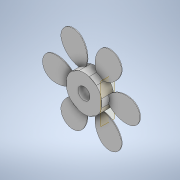
# Autodesk Inventor part: Fan
Saved by Autodesk Inventor 2022 (Build 260153000, 153)
## iProperties
Created: 2021-07-12
Part Number: Fan
Material: Generic
Document SubType Name: Modeling
Designer: Mike
Density: 1 g/cm^3
Appearance: Default
Author: Mike
Autodesk Inventor part; units mm, degrees
ref_plane "XZ Plane" through (0, 0, 0) normal (0, 1, 0) x (-1, 0, 0)
ref_plane "XY Plane" through (0, 0, 0) normal (0, 0, 1) x (1, 0, 0)
sketch "Sketch1" plane through (0, 0, 0) normal (0, 0, 1) x (1, 0, 0)
  circle A0 centre (0, 0) radius 7.5
  circle A1 centre (0, 0) radius 2.5
  dimension "d0" = 15
  dimension "d1" = 5
  constraints: 2 centre point, 2 coincident
  measures "d0" diameter of A0
  measures "d1" diameter of A1
extrude "Extrusion1" add sketch "Sketch1" against normal blind 5
ref_plane "Work Plane1" through (7.3, 0, 0) normal (1, 0, 0) x (0, 1, 0)
sketch "Sketch2" plane through (7.3, 0, 0) normal (1, 0, 0) x (0, 1, 0)
  line L0 (1.7003, -3.2966) -> (-1.6964, -3.2966)
  line L1 (-1.6964, -3.2966) -> (-1.6964, -3.0015)
  line L2 (-1.6964, -3.0015) -> (1.7003, -3.0015)
  line L3 (1.7003, -3.0015) -> (1.7003, -3.2966)
  point P0 (0, 0)
  dimension "d5" = 3.3967
  dimension "d6" = 0.2951
  dimension "d7" = 1.7003
  dimension "d8" = 3.0015
  constraints: 8 end point, 2 parallel, 1 horizontal, 1 perpendicular
  measures "d5" distance between parallel lines of L3 L1
  measures "d6" distance between parallel lines of L0 L2
  measures "d7" distance from line of point (0, 0) L3
  measures "d8" distance from line of point (0, 0) L2
extrude "Extrusion2" add sketch "Sketch2" along normal blind 20
sketch "Sketch3" plane through (7.3047, 1.7003, -3.0015) normal (0, 1, 0) x (1, 0, 0)
  line L0 (19.9953, 0) -> (19.9953, 0.2951) projected
  line L1 (-0.0143, 0) -> (19.9953, 0)
  line L2 (19.9953, 0) -> (19.9953, 0.2951)
  line L3 (19.9953, 0.2951) -> (-0.0143, 0.2951)
  line L4 (-0.0143, 0.2951) -> (-0.0143, 0)
  point P0 (-7.3047, -3.0015)
  constraints: 8 end point, 2 parallel, 1 horizontal, 1 perpendicular
extrude "Extrusion3" add sketch "Sketch3" along normal blind 10 and the other way blind 20
sketch "Sketch4" plane through (27.3, 11.7003, -3.2966) normal (0, 0, -1) x (-1, 0, 0)
  circle A0 centre (27.3, -11.7003) radius 7.5 projected
  arc A1 (24.9034, -4.5935) -> (24.9034, -4.5935) centre (30.4717, -11.6954) ccw
  arc A2 (11.0151, -6.7908) -> (11.0151, -16.6097) centre (11.9624, -11.7003) ccw
  arc A3 (11.0151, -16.6097) -> (19.9875, -13.3669) centre (12.7805, -7.4601) ccw
  line L0 (27.3, -11.7003) -> (11.9624, -11.7003) construction
  arc A4 (19.9875, -10.0336) -> (11.0151, -6.7908) centre (12.7805, -15.9404) ccw
  line L1 (20.0095, 0) -> (0, 0) projected
  line L2 (20.0095, -30) -> (20.0095, -13.4607) projected
  line L3 (0, 0) -> (20.0095, 0)
  line L4 (20.0095, 0) -> (20.0095, -30)
  line L5 (20.0095, -30) -> (0, -30)
  line L6 (0, -30) -> (0, 0)
  point P0 (20.0095, -9.9398)
  dimension "d15" = 10
  dimension "d16" = 9.0245
  dimension "d17" = 9.3183
  dimension "d18" = 0.0049
  dimension "d19" = 7.1068
  dimension "d20" = 1.6667
  dimension "d21" = 4.2401
  constraints: 11 point on circle, 10 end point, 4 centre point, 3 symmetric about line, 2 horizontal, 2 parallel, 1 perpendicular, 1 tangent, 1 other
  measures "d15" diameter of A2
  measures "d16" radius of A1
  measures "d17" radius of A3
  measures "d18" distance from line of A1.centre L0
  measures "d19" distance from line of A0.start L0
  measures "d20" distance from line of A4.start L0
  measures "d21" distance from line of A3.centre L0
extrude "Extrusion4" cut sketch "Sketch4" against normal up to next contours A4 A2 A3 A0 L2 L5 L6 L1 L4
split body "Split5" result two bodies by plane through (7.3, 0, 0) normal (1, 0, 0) first body at (17.2545, 1.061, -3.1966)
pattern_circular "Circular Pattern4" count 6 over 360 about axis through (0, 0, -10) along (0, 0, 1) bodies 2
body "Solid4"
body "Solid5"
body "Solid6"
body "Solid7"
